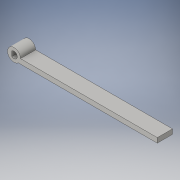
# Autodesk Inventor part: Rotator2
Saved by Autodesk Inventor 2016 SP1 (Build 200210100, 210)
## iProperties
Created: 2016-04-13
Part Number: Rotator2
Material: Generic
Document SubType Name: Modeling
Designer: schiu30
Density: 1 g/cm^3
Appearance: Default
Author: schiu30
Autodesk Inventor part; units mm, degrees
ref_plane "YZ Plane" through (0, 0, 0) normal (1, 0, 0) x (0, 1, 0)
ref_plane "XZ Plane" through (0, 0, 0) normal (0, 1, 0) x (-1, 0, 0)
ref_plane "XY Plane" through (0, 0, 0) normal (0, 0, 1) x (1, 0, 0)
sketch "Sketch1" plane through (0, 0, 0) normal (0, 0, 1) x (1, 0, 0)
  arc A0 (-1.325, -1.5313) -> (-1.325, 1.5313) centre (0, 0) ccw
  line L0 (-1.325, -1.5313) -> (-1.325, 1.5313)
  arc A1 (4, 0) -> (2.6774, -2.9718) centre (0, 0) ccw
  line L1 (2.6774, -2.9718) -> (88.9, -2.9718)
  line L2 (88.9, -2.9718) -> (88.9, 0)
  line L3 (88.9, 0) -> (4, 0)
  dimension "d0" = 4.05
  dimension "d2" = 8
  dimension "d3" = 3.35
  dimension "d5" = 88.9
  dimension "d7" = 2.9718
  dimension "d8" = 84.9
  constraints: 8 end point, 4 point on circle, 2 centre point, 2 coincident, 1 horizontal, 1 parallel, 1 perpendicular, 1 vertical
  measures "d0" diameter of A0
  measures "d2" diameter of A1
  measures "d5" distance of A1.centre L2.end
  measures "d7" distance of L1.end L2.end
  measures "d8" distance of L2.end L3.end
extrude "Extrusion1" add sketch "Sketch1" along normal blind 9.398
body "Solid1"
